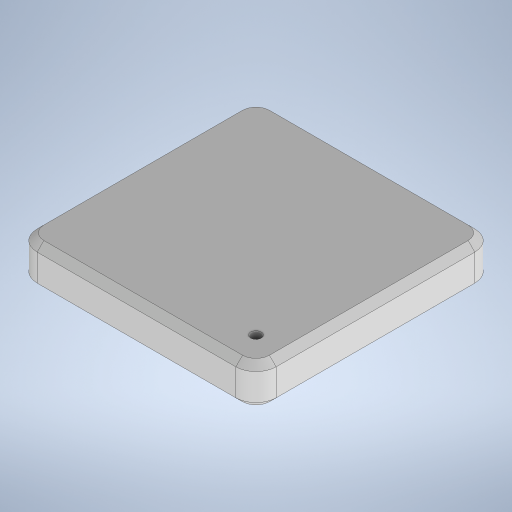
# Autodesk Inventor part: plate
Saved by Autodesk Inventor 2024.3 (Build 283343000, 343)
## iProperties
Created: 2026-03-13
Part Number: plate
Material: Generico
Document SubType Name: Modeling
Designer: chris
Density: 1 g/cm^3
Appearance: Default
Author: chris
Autodesk Inventor part; units mm, degrees
ref_plane "YZ Plane" through (0, 0, 0) normal (1, 0, 0) x (0, 1, 0)
ref_plane "XZ Plane" through (0, 0, 0) normal (0, 1, 0) x (-1, 0, 0)
ref_plane "XY Plane" through (0, 0, 0) normal (0, 0, 1) x (1, 0, 0)
sketch "Schizzo1" plane through (0, 0, 0) normal (0, 0, 1) x (1, 0, 0)
  line L0 (0.089, 0.089) -> (-0.089, 0.089)
  line L1 (-0.089, 0.089) -> (-0.089, -0.089)
  line L2 (-0.089, -0.089) -> (0.089, -0.089)
  line L3 (0.089, -0.089) -> (0.089, 0.089)
  line L4 (0.089, 0.089) -> (-0.089, -0.089) construction
  line L5 (-0.089, 0.089) -> (0.089, -0.089) construction
  point P0 (0, 0)
  dimension "d0" = 0.178
  dimension "d1" = 0.178
  constraints: 12 end point, 2 midpoint, 2 parallel, 1 horizontal, 1 perpendicular
  measures "d0" distance of L0.start L0.end
  measures "d1" distance of L0.end L1.end
extrude "Estrusione1" add sketch "Schizzo1" along normal blind 0.03
sketch "Schizzo2" plane through (0, 0, 0.03) normal (0, 0, 1) x (1, 0, 0)
  line L0 (-0.089, 0.089) -> (-0.089, -0.089) construction
  line L1 (-0.089, -0.089) -> (0.089, -0.089) construction
  line L2 (0.089, -0.089) -> (0.089, 0.089) construction
  line L3 (0.089, 0.089) -> (-0.089, 0.089) construction
  circle A0 centre (0.066, 0.066) radius 0.004
  point P0 (0, 0)
  dimension "d4" = 0.023
  dimension "d5" = 0.023
  dimension "d6" = 0.008
  constraints: 1 centre point
  measures "d4" distance from line of L3 A0.centre
  measures "d5" distance from line of L2 A0.centre
  measures "d6" diameter of A0
extrude "Estrusione2" cut sketch "Schizzo2" against normal through all
fillet "Raccordo1" radius 0.015 4 edges at (0.089, 0.089, 0.015) (-0.089, 0.089, 0.015) (0.089, -0.089, 0.015) (-0.089, -0.089, 0.015)
chamfer "Smusso1" distance 0.005 angle 45 16 edges at (0, 0.089, 0.03) (-0.0846, 0.0846, 0.03) (-0.089, 0, 0.03) (-0.0846, -0.0846, 0.03) (0, -0.089, 0.03) (0.0846, -0.0846, 0.03) (0.089, 0, 0.03) (0.0846, 0.0846, 0.03) (0, 0.089, 0) (-0.0846, 0.0846, 0) (-0.089, 0, 0) (-0.0846, -0.0846, 0) (0, -0.089, 0) (0.0846, -0.0846, 0) (0.089, 0, 0) (0.0846, 0.0846, 0)
